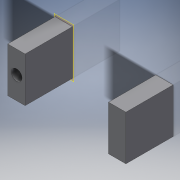
# Autodesk Inventor part: bracket
Saved by Autodesk Inventor 2019 (Build 230136000, 136)
## iProperties
Created: 2020-07-29
Part Number: bracket
Material: Generic
Document SubType Name: Modeling
Designer: Ian
Density: 1 g/cm^3
Appearance: Default
Author: Ian
Autodesk Inventor part; units mm, degrees
ref_plane "YZ Plane" through (0, 0, 0) normal (1, 0, 0) x (0, 1, 0)
ref_plane "Work Plane1" through (0, 0, 0) normal (0, 0, 1) x (1, 0, 0)
sketch "Sketch1" plane through (0, 0, 0) normal (0, 0, 1) x (1, 0, 0)
  line L0 (5, 0) -> (5, 12.5) projected
  line L1 (0, 12.5) -> (5, 12.5) projected
  line L2 (0, 0) -> (0, 12.5) projected
  line L3 (0, 0) -> (5, 0) projected
  line L4 (28, 12.5) -> (28, 0) projected
  line L5 (28, 0) -> (33, 0) projected
  line L6 (33, 0) -> (33, 12.5) projected
  line L7 (28, 12.5) -> (33, 12.5) projected
  line L8 (4.85, 12.5) -> (4.85, 0)
  line L9 (28.15, 0) -> (28.15, 12.5)
  dimension "d5" = 0.15
  dimension "d6" = 0.15
  constraints: 4 end point, 4 point on line
  measures "d5" distance between parallel lines of L0 L8
  measures "d6" distance between parallel lines of L4 L9
ref_plane "Work Plane2" through (12, 13.25, 13.2) normal (0, 0, 1) x (1, 0, 0)
extrude "Extrusion1" add sketch "Sketch1" along normal up to surface (13.2 mm away) contours L3 L2 L1 L8 | L7 L6 L5 L9
sketch "Sketch2" plane through (0, 0, 0) normal (0, 0, -1) x (-1, 0, 0)
  circle A0 centre (-2.5, 6.25) radius 1.5
  line L0 (-4.85, 12.5) -> (0, 12.5) construction
  line L1 (-2.5, 12.5) -> (-2.5, 0) construction
  point P0 (0, 0)
  point P1 (-5, 12.5)
  point P2 (-2.5, 6.25)
  dimension "d2" = 3
  constraints: 2 end point, 1 centre point, 1 coincident, 1 midpoint, 1 point on line, 1 vertical
  measures "d2" diameter of A0
extrude "Extrusion2" cut sketch "Sketch2" against normal through all
ref_plane "Work Plane3" through (28.15, 12.65, 0) normal (0, 1, 0) x (1, 0, 0)
sketch "Sketch3" plane through (28.15, 12.65, 0) normal (0, 1, 0) x (1, 0, 0)
  line L0 (4.85, 0) -> (4.85, -13.2) projected
  line L1 (4.85, -9.7385) -> (-28.15, -9.7385)
  line L2 (-28.15, -9.7385) -> (-28.15, -4.1615)
  line L3 (-28.15, -4.1615) -> (4.85, -4.1615)
  line L4 (4.85, -4.1615) -> (4.85, -9.7385)
  line L5 (-9.637, -4.1615) -> (-3.163, -4.1615) projected
  line L6 (-3.163, -9.7385) -> (-9.637, -9.7385) projected
  line L7 (-28.15, -13.2) -> (-23.3, -13.2) projected
  line L8 (-23.3, 0) -> (-23.3, -13.2) projected
  line L9 (-23.3, 0) -> (-28.15, 0) projected
  line L10 (-28.15, 0) -> (-28.15, -13.2) projected
  point P0 (-28.15, 0)
  constraints: 8 end point, 3 collinear, 2 parallel, 1 horizontal, 1 perpendicular, 1 point on line
extrude "Extrusion3" add sketch "Sketch3" along normal blind 2 contours L0 L1 L8 L3 | L8 L1 L2 L3
sketch "Sketch4" plane through (28.15, 12.65, 0) normal (0, -1, 0) x (1, 0, 0)
  line L0 (4.85, 9.7385) -> (-28.15, 9.7385) projected
  line L1 (-28.15, 9.7385) -> (-28.15, 4.1615) projected
  line L2 (-28.15, 4.1615) -> (4.85, 4.1615) projected
  line L3 (4.85, 4.1615) -> (4.85, 9.7385) projected
  line L4 (-23.3, 13.2) -> (-28.15, 13.2) projected
  line L5 (-28.15, 0) -> (-28.15, 13.2) projected
  line L6 (-28.15, 0) -> (-23.3, 0) projected
  line L7 (-23.3, 0) -> (-23.3, 13.2) projected
  line L8 (4.85, 13.2) -> (0, 13.2) projected
  line L9 (0, 0) -> (0, 13.2) projected
  line L10 (0, 0) -> (4.85, 0) projected
  line L11 (4.85, 0) -> (4.85, 13.2) projected
  line L12 (-28.15, 9.7385) -> (4.85, 9.7385) projected
  line L13 (-28.15, 4.1615) -> (-23.3, 4.1615)
  line L14 (-23.3, 4.1615) -> (-23.3, 9.7385)
  line L15 (-23.3, 9.7385) -> (-28.15, 9.7385)
  line L16 (-28.15, 9.7385) -> (-28.15, 4.1615)
  line L17 (4.85, 9.7385) -> (4.85, 4.1615) projected
  line L18 (0, 9.7385) -> (4.85, 9.7385)
  line L19 (4.85, 9.7385) -> (4.85, 4.1615)
  line L20 (4.85, 4.1615) -> (0, 4.1615)
  line L21 (0, 4.1615) -> (0, 9.7385)
  point P0 (-28.15, 0)
  constraints: 16 end point, 4 parallel, 4 point on line, 2 horizontal, 2 perpendicular
extrude "Extrusion4" add sketch "Sketch4" along normal up to surface (0.15 mm away) contours L3 L2 L9 L0 | L7 L2 L1 L0
sketch "Sketch5" plane through (0, 0, 0) normal (0, -1, 0) x (1, 0, 0)
  line L0 (4.85, 13.2) -> (0, 13.2) projected
  line L1 (0, 0) -> (0, 13.2) projected
  line L2 (0, 0) -> (4.85, 0) projected
  line L3 (4.85, 0) -> (4.85, 13.2) projected
  line L4 (33, 13.2) -> (28.15, 13.2) projected
  line L5 (28.15, 0) -> (28.15, 13.2) projected
  line L6 (28.15, 0) -> (33, 0) projected
  line L7 (33, 0) -> (33, 13.2) projected
  point P0 (0, 0)
extrude "Extrusion5" add sketch "Sketch5" along normal blind 0.15
sketch "Sketch6" plane through (0, -0.15, 0) normal (0, -1, 0) x (1, 0, 0)
  line L0 (33, 0) -> (28.15, 0) projected
  line L1 (0, 9.7385) -> (0, 13.2) projected
  line L2 (33, 0) -> (0, 0)
  line L3 (0, 0) -> (0, 13.2)
  line L4 (0, 13.2) -> (33, 13.2)
  line L5 (33, 13.2) -> (33, 0)
  point P0 (0, 0)
  constraints: 8 end point, 2 parallel, 1 horizontal, 1 perpendicular
extrude "Extrusion6" add sketch "Sketch6" along normal blind 3
sketch "Sketch7" plane through (28.15, 14.65, 0) normal (0, 1, 0) x (1, 0, 0)
  line L0 (-28.15, -4.1615) -> (-23.3, -4.1615) projected
  line L1 (-23.3, 0) -> (-23.3, -4.1615) projected
  line L2 (-23.3, 0) -> (-28.15, 0) projected
  line L3 (-28.15, 0) -> (-28.15, -4.1615) projected
  line L4 (-23.3, -9.7385) -> (-28.15, -9.7385) projected
  line L5 (-28.15, -9.7385) -> (-28.15, -13.2) projected
  line L6 (-28.15, -13.2) -> (-23.3, -13.2) projected
  line L7 (-23.3, -9.7385) -> (-23.3, -13.2) projected
  line L8 (0, -4.1615) -> (4.85, -4.1615) projected
  line L9 (4.85, 0) -> (4.85, -4.1615) projected
  line L10 (4.85, 0) -> (0, 0) projected
  line L11 (0, 0) -> (0, -4.1615) projected
  line L12 (-16.2355, -12.1401) -> (3.4355, -12.1401) projected
  line L13 (4.85, -9.7385) -> (0, -9.7385) projected
  line L14 (0, -9.7385) -> (0, -13.2) projected
  line L15 (0, -13.2) -> (4.85, -13.2) projected
  line L16 (4.85, -9.7385) -> (4.85, -13.2) projected
  point P0 (-28.15, 0)
extrude "Extrusion7" add sketch "Sketch7" against normal up to surface (2.15 mm away)
fillet "Fillet1" radius 3 4 edges at (4.85, 13.65, 9.7385) (4.85, 13.65, 4.1615) (28.15, 13.65, 4.1615) (28.15, 13.65, 9.7385)
sketch "Sketch8" plane through (28.15, 14.65, 13.2) normal (0, 0, 1) x (1, 0, 0)
  circle A0 centre (-25.65, -8.4) radius 1.5 projected
  line L0 (-28.15, -17.8) -> (-28.15, 0) projected
  line L1 (4.85, -17.8) -> (-28.15, -17.8) projected
  line L2 (4.85, 0) -> (4.85, -17.8) projected
  line L3 (0, 0) -> (4.85, 0) projected
  line L4 (0, -14.8) -> (0, 0) projected
  line L5 (-23.3, -14.8) -> (0, -14.8) projected
  line L6 (-23.3, 0) -> (-23.3, -14.8) projected
  line L7 (-28.15, 0) -> (-23.3, 0) projected
  point P0 (-28.15, -14.65)
extrude "Extrusion8" add sketch "Sketch8" along normal blind 0.15
sketch "Sketch9" plane through (28.15, 14.65, 13.35) normal (0, 0, 1) x (1, 0, 0)
  circle A0 centre (-6.4, 8.35) radius 2.25 projected
  circle A1 centre (-6.4, 8.35) radius 2.45
  line L0 (-28.15, -2.15) -> (-23.15, -2.15) projected
  circle A2 centre (-25.65, -8.4) radius 1.5 projected
  line L1 (-28.15, 0) -> (-28.15, -17.8) projected
  line L2 (-28.15, -17.8) -> (4.85, -17.8) projected
  line L3 (4.85, -17.8) -> (4.85, 0) projected
  line L4 (4.85, 0) -> (0, 0) projected
  line L5 (0, 0) -> (0, -14.8) projected
  line L6 (0, -14.8) -> (-23.3, -14.8) projected
  line L7 (-23.3, -14.8) -> (-23.3, 0) projected
  line L8 (-23.3, 0) -> (-28.15, 0) projected
  line L9 (-23.3, 0) -> (-28.15, 0) projected
  line L10 (-28.15, 0) -> (-23.3, 0)
  line L11 (-23.3, 0) -> (-23.3, 12.35)
  line L12 (-23.3, 12.35) -> (-28.15, 12.35)
  line L13 (-28.15, 12.35) -> (-28.15, 0)
  line L14 (4.85, 0) -> (0, 0) projected
  line L15 (0, 0) -> (4.85, 0)
  line L16 (4.85, 0) -> (4.85, 12.35)
  line L17 (4.85, 12.35) -> (0, 12.35)
  line L18 (0, 12.35) -> (0, 0)
  line L19 (-28.15, 12.35) -> (4.85, 12.35)
  line L20 (4.85, 12.35) -> (4.85, 4.35)
  line L21 (4.85, 4.35) -> (-28.15, 4.35)
  line L22 (-28.15, 4.35) -> (-28.15, 12.35)
  line L23 (4.85, -17.8) -> (4.85, 0) projected
  line L24 (-23.3, -14.8) -> (-23.3, 0) projected
  point P0 (-28.15, -14.65)
  dimension "d21" = 0.2
  dimension "d22" = 4
  dimension "d23" = 4
  constraints: 24 end point, 6 parallel, 3 collinear, 3 horizontal, 3 perpendicular, 1 centre point, 1 point on line
  measures "d21" radial gap between concentric circles of A0 A1
  measures "d22" distance from line of A0.centre L19
  measures "d23" distance from line of A0.centre L21
extrude "Extrusion9" add sketch "Sketch9" along normal blind 3 contours L1 L8 L7 L0 | L0 L7 L6 L5 L4 L3 L2 L1 | L13 L21 L11 L8 | L13 L12 L11 L21 | L11 L19 L18 L21 | L4 L18 L21 L16 | L18 L17 L16 L21
fillet "Fillet2" radius 3 2 edges at (30.575, 14.65, 13.35) (2.425, 14.65, 13.35)
fillet "Fillet3" radius 3 2 edges at (33, 27, 14.85) (0, 27, 14.85)
sketch "Sketch11" plane through (0, -3.15, 0) normal (-1, 0, 0) x (0, 0, 1)
  line L0 (13.35, 27.15) -> (16.35, 27.15) projected
  line L1 (13.35, 27.15) -> (13.35, 20.8) projected
  arc A0 (10.35, 17.8) -> (13.35, 20.8) centre (10.35, 20.8) ccw projected
  line L2 (0, 17.8) -> (10.35, 17.8) projected
  line L3 (0, 17.8) -> (0, 0) projected
  line L4 (0, 0) -> (16.35, 0) projected
  line L5 (16.35, 27.15) -> (16.35, 0) projected
  line L6 (0, 0) -> (16.35, 0)
  line L7 (16.35, 0) -> (16.35, -24.5)
  line L8 (16.35, -24.5) -> (0, -24.5)
  line L9 (0, -24.5) -> (0, 0)
  line L10 (-17.95, 11.4767) -> (-11.95, 11.4767) projected
  line L11 (-11.95, 11.4767) -> (-11.95, 7.3233) projected
  line L12 (-11.95, 7.3233) -> (-17.95, 7.3233) projected
  line L13 (-17.95, 7.3233) -> (-17.95, -24.5) projected
  line L14 (-17.95, -24.5) -> (0, -24.5) projected
  line L15 (0, -24.5) -> (0, 3.15) projected
  line L16 (-2.5, 3.15) -> (0, 3.15) projected
  line L17 (-2.5, 15.65) -> (-2.5, 3.15) projected
  line L18 (-2.5, 15.65) -> (0, 15.65) projected
  line L19 (0, 17.8) -> (0, 15.65) projected
  line L20 (0, 17.8) -> (-11.95, 17.8) projected
  arc A1 (-14.95, 20.8) -> (-11.95, 17.8) centre (-11.95, 20.8) ccw projected
  line L21 (-14.95, 27.15) -> (-14.95, 20.8) projected
  line L22 (-14.95, 27.15) -> (-17.95, 27.15) projected
  line L23 (-17.95, 27.15) -> (-17.95, 11.4767) projected
  constraints: 8 end point, 2 parallel, 1 collinear, 1 horizontal, 1 perpendicular
extrude "Extrusion10" add sketch "Sketch11" against normal blind 5 contours L7 L8 L9 L4
sketch "Sketch12" plane through (28.15, 14.65, 16.35) normal (0, 0, 1) x (1, 0, 0)
  line L0 (-23.15, -17.8) -> (-23.15, -37.3) projected
  line L1 (-23.15, -17.8) -> (4.85, -17.8) projected
  line L2 (4.85, -17.8) -> (4.85, -14.65) projected
  line L3 (4.85, -14.65) -> (0, -14.65) projected
  line L4 (0, -14.65) -> (0, -14.8) projected
  line L5 (0, -14.8) -> (-23.3, -14.8) projected
  line L6 (-23.3, -14.8) -> (-23.3, -14.65) projected
  line L7 (-23.3, -14.65) -> (-28.15, -14.65) projected
  line L8 (-28.15, -42.3) -> (-28.15, -14.65) projected
  line L9 (-28.15, -42.3) -> (4.85, -42.3) projected
  line L10 (4.85, -42.3) -> (4.85, -37.3) projected
  line L11 (-23.15, -37.3) -> (4.85, -37.3) projected
  line L12 (-23.15, -17.8) -> (-23.15, -42.3) projected
  line L13 (-23.15, -37.3) -> (-23.15, -42.3)
  constraints: 2 end point, 1 vertical
ref_plane "Work Plane4" through (0, -27.65, 0) normal (0, 0, 1) x (1, 0, 0)
extrude "Extrusion11" add sketch "Sketch12" against normal up to surface (16.35 mm away) contours L11 L10 L9 L12
sketch "Sketch13" plane through (0, 0, 0) normal (0, 0, -1) x (-1, 0, 0)
  circle A0 centre (-30.5, -25.15) radius 1.5
  circle A1 centre (-2.5, -25.15) radius 1.5
  circle A2 centre (-16.5, -25.15) radius 1.5
  line L0 (-30.5, -25.15) -> (-16.5, -25.15) construction
  line L1 (-16.5, -25.15) -> (-2.5, -25.15) construction
  line L2 (-33, -22.65) -> (-33, -27.65) construction
  line L3 (-5, -22.65) -> (-33, -22.65) construction
  line L4 (0, 14.65) -> (0, -27.65) construction
  point P0 (0, 0)
  dimension "d33" = 3
  dimension "d34" = 3
  dimension "d36" = 3
  dimension "d37" = 2.5
  dimension "d38" = 2.5
  dimension "d39" = 2.5
  constraints: 4 end point, 3 centre point, 2 collinear, 1 horizontal
  measures "d33" diameter of A1
  measures "d34" diameter of A0
  measures "d36" diameter of A2
  measures "d37" distance from line of L0.start L2
  measures "d38" distance between parallel lines of L3 L0
  measures "d39" distance from line of L4 L1.end
extrude "Extrusion12" add sketch "Sketch13" along normal blind 2
fillet "Fillet4" radius 0.25 3 edges at (32, -25.15, -2) (18, -25.15, -2) (4, -25.15, -2)
body "Solid1"
